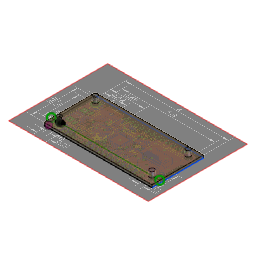
Enclosure v1 (Autodesk Fusion 360 design; units mm, degrees)
Autodesk Fusion 360 part; units mm, degrees
sketch "Sketch3" plane through (0, 0, 0) normal (0, 0, 1) x (1, 0, 0)
  line L0 (0, 0) -> (50.8, 0) construction
  line L1 (50.8, 0) -> (50.8, 22.86) construction
  line L2 (50.8, 22.86) -> (0, 22.86) construction
  line L3 (0, 22.86) -> (0, 0) construction
  line L4 (25.4, 22.86) -> (25.4, 0) construction
  line L5 (0, 11.43) -> (50.8, 11.43) construction
  line L6 (-1.27, -1.27) -> (52.07, -1.27)
  line L7 (52.07, -1.27) -> (52.07, 24.13)
  line L8 (52.07, 24.13) -> (-1.27, 24.13)
  line L9 (-1.27, 24.13) -> (-1.27, -1.27)
  dimension "d4" = 1.27
extrude "Extrude2" add sketch "Sketch3" along normal blind 1.27 makes body 1
sketch "Sketch4" plane through (0, 0, 1.27) normal (0, 0, 1) x (-1, 0, 0)
  line L0 (1.27, -24.13) -> (1.27, 1.27)
  line L1 (1.27, 1.27) -> (-52.07, 1.27)
  line L2 (-52.07, 1.27) -> (-52.07, -24.13)
  line L3 (-52.07, -24.13) -> (1.27, -24.13)
  circle A0 centre (-2.54, -2.54) radius 1.27
  dimension "d7" = 2.54
  measures "d7" diameter of A0
ref_plane "WorkPlane4" through (0, 2.54, 0) normal (0, 1, 0) x (0, 0, 1)
sketch "Sketch7" plane through (0, 2.54, 0) normal (0, 1, 0) x (1, 0, 0)
  line L0 (52.07, -1.27) -> (-1.27, -1.27)
  line L1 (2.54, -1.27) -> (3.81, -1.27)
  line L2 (3.81, -1.27) -> (3.683, -3.8506)
  line L3 (3.683, -3.8506) -> (2.54, -3.8506)
  line L4 (2.54, -3.8506) -> (2.54, -1.27)
  dimension "d18" = 1.143
  dimension "d19" = 1.27
  dimension "d20" = 2.5806
revolve "Revolve2" add sketch "Sketch7" angle 360 about axis through (2.54, 2.54, -52.07) along (0, 0, 1) separate body makes body 2
pattern_linear "R-Pattern1" count 2 spacing 45.72 along (1, 0, 0) count 2 spacing 17.78 along (0, 1, 0) of bodies 2 makes body 3 at (47.4814, 3.5164, 1.7001) makes body 4 at (1.2912, 20.32, 1.7001) makes body 5 at (47.4814, 21.2964, 1.7001)
ref_plane "WorkPlane2" through (0, 2.54, 0) normal (0, 1, 0) x (0, 0, 1)
revolve "Revolve1" [rolled back] along angle 360 against angle 0
sketch "Sketch6" plane through (0, 0, 0) normal (0, 1, 0) x (1, 0, 0)
extrude "Extrude3" [rolled back] along distance 4.7625 taper angle 0
hole "Hole1" [rolled back] hole depth 6.35 hole diameter 1.9304 tip angle 180
equation "d13 = ( 3 / 16 ) * 1 in"
equation "d15 = ( 1 / 4 ) * 1 in"
equation "d18 = ( 0.09 / 2 ) * 1 in"
equation "d19 = ( 0.1 / 2 ) * 1 in"
equation "d20 = ( 4 * 0.0254 ) * 1 in"
